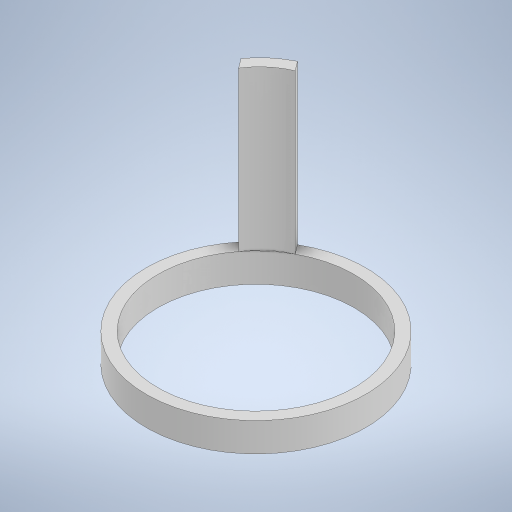
# Autodesk Inventor part: scoringelement2
Saved by Autodesk Inventor 2023 (Build 270158000, 158)
## iProperties
Created: 2022-11-10
Part Number: scoringelement2
Material: Generic
Document SubType Name: Modeling
Designer: myan
Density: 1 g/cm^3
Appearance: Default
Author: myan
Autodesk Inventor part; units mm, degrees
ref_plane "YZ Plane" through (0, 0, 0) normal (1, 0, 0) x (0, 1, 0)
ref_plane "XZ Plane" through (0, 0, 0) normal (0, 1, 0) x (-1, 0, 0)
ref_plane "XY Plane" through (0, 0, 0) normal (0, 0, 1) x (1, 0, 0)
sketch "Sketch1" plane through (0, 0, 0) normal (0, 1, 0) x (-1, 0, 0)
  circle A0 centre (0, 0) radius 48.26
  circle A1 centre (0, 0) radius 43.18
  dimension "d0" = 96.52
  dimension "d1" = 86.36
  constraints: 2 centre point, 2 coincident
  measures "d0" diameter of A0
  measures "d1" diameter of A1
extrude "Extrusion1" add sketch "Sketch1" along normal blind 12.7
sketch "Sketch2" plane through (0, 12.7, 0) normal (0, 1, 0) x (1, 0, 0)
  circle A0 centre (0, 0) radius 48.26 projected
  arc A1 (-23.7559, 42.0082) -> (-37.2641, 30.6662) centre (-7.0461, 8.3919) ccw
  circle A2 centre (0, 0) radius 43.18 projected
  arc A3 (-20.6666, 37.9131) -> (-34.1068, 26.4809) centre (-9.1261, 10.7291) ccw
  line L0 (-34.1068, 26.4809) -> (-37.2641, 30.6662)
  line L1 (-23.7559, 42.0082) -> (-20.6666, 37.9131)
  constraints: 8 point on circle, 4 end point, 2 centre point, 1 parallel
extrude "Extrusion2" add sketch "Sketch2" along normal blind 69.85 contours L1 A3 L0 A0 | A0 A1
body "Solid1"
